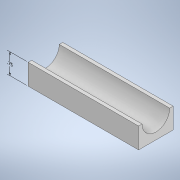
# Autodesk Inventor part: Ball Ramp - Goldberg
Saved by Autodesk Inventor 2021 (Build 250183000, 183)
## iProperties
Created: 2021-02-16
Part Number: Ball Ramp - Goldberg
Material: Generic
Document SubType Name: Modeling
Designer: david
Density: 1 g/cm^3
Appearance: Default
Author: david
Autodesk Inventor part; units mm, degrees
ref_plane "YZ Plane" through (0, 0, 0) normal (1, 0, 0) x (0, 1, 0)
ref_plane "XZ Plane" through (0, 0, 0) normal (0, 1, 0) x (-1, 0, 0)
ref_plane "XY Plane" through (0, 0, 0) normal (0, 0, 1) x (1, 0, 0)
sketch "Sketch1" plane through (0, 0, 0) normal (1, 0, 0) x (0, 1, 0)
  line L0 (19.05, -2.1167) -> (0, -2.1167)
  line L1 (0, -2.1167) -> (0, -33.8667)
  line L2 (0, -33.8667) -> (19.05, -33.8667)
  arc A0 (19.05, -5.2917) -> (19.05, -30.6917) centre (19.05, -17.9917) ccw
  line L3 (19.05, -33.8667) -> (19.05, -30.6917)
  line L4 (19.05, -5.2917) -> (19.05, -2.1167)
  point P0 (0, 0)
  dimension "d0" = 12.7
  dimension "d1" = 19.05
  dimension "d2" = 31.75
  dimension "d3" = 19.05
  dimension "d4" = 19.05
  constraints: 10 end point, 3 parallel, 2 point on circle, 1 centre point, 1 horizontal, 1 perpendicular
  measures "d0" radius of A0
  measures "d1" distance of L0.start L0.end
  measures "d2" distance of L0.end L1.end
  measures "d3" distance of L1.end L2.end
  measures "d4" distance from line of L1 A0.centre
extrude "Extrusion1" add sketch "Sketch1" along normal blind 101.6
body "Solid1"
